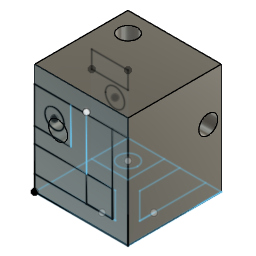
cornerpiece_test1 (Autodesk Fusion 360 design; units mm, degrees)
Autodesk Fusion 360 part; units mm, degrees
note: some values were not read from the file. Set by a fixed rule: which sketch regions a step uses.
sketch "Skizze1" plane through (0, 0, 0) normal (0, 0, 1) x (1, 0, 0)
  line L0 (4.1176, 5.2824) -> (204.1176, 5.2824)
  line L1 (204.1176, 5.2824) -> (204.1176, 205.2824)
  line L2 (204.1176, 205.2824) -> (4.1176, 205.2824)
  line L3 (4.1176, 205.2824) -> (4.1176, 5.2824)
  line L4 (204.1176, 48.8824) -> (207.3176, 48.8824)
  line L5 (207.3176, 48.8824) -> (207.3176, 13.2824)
  line L6 (207.3176, 13.2824) -> (204.1176, 13.2824)
  line L7 (204.1176, 13.2824) -> (204.1176, 48.8824)
  line L8 (196.1176, 13.2824) -> (207.1176, 13.2824)
  line L9 (207.1176, 13.2824) -> (207.1176, 2.2824)
  line L10 (207.1176, 2.2824) -> (196.1176, 2.2824)
  line L11 (196.1176, 2.2824) -> (196.1176, 13.2824)
  circle A0 centre (202.6176, 6.7824) radius 1
  line L12 (202.1176, 5.2824) -> (204.1176, 7.2824)
  dimension "top_w" = 200
  dimension "top_l" = 200
  dimension "d12" = 3.2
  dimension "d13" = 35.6
  dimension "d14" = 11
  dimension "d15" = 11
  dimension "d17" = 2
  dimension "d18" = 1.5
  dimension "d19" = 1.5
  dimension "d23" = 3
  dimension "d24" = 3
  dimension "d28" = 2
  dimension "d29" = 2
  constraint horizontal L0
  constraint vertical L1
  constraint horizontal L2
  constraint vertical L3
  constraint horizontal L4
  constraint vertical L5
  constraint horizontal L6
  constraint vertical L7
  constraint horizontal L8
  constraint vertical L9
  constraint horizontal L10
  constraint vertical L11
  constraint coincident L6.end L8
  constraint coincident L1 L6.end
  constraint coincident L0 L12.start
  constraint coincident L1 L12.end
  measures "top_w" distance of L0.start L0.end
  measures "top_l" distance of L0.start L2.end
  measures "d12" distance of L4.start L4.end
  measures "d13" distance of L4.start L6.end
  measures "d14" distance of L8.start L8.end
  measures "d15" distance of L8.start L10.end
  measures "d17" diameter of A0
  measures "d18" horizontal distance of L0.end A0.centre
  measures "d19" vertical distance of L0.end A0.centre
  measures "d23" horizontal distance of L0.end L9.end
  measures "d24" vertical distance of L0.end L9.end
  measures "d28" distance of L0.end L12.end
  measures "d29" distance of L0.end L12.start
sketch "Skizze2" plane through (0, 0, 0) normal (0, 0, 1) x (1, 0, 0)
  line L0 (17.1763, 11.0643) -> (17.1763, 0.2643)
  line L1 (6.3763, 0.2643) -> (6.3763, 11.0643)
  line L2 (6.3763, 11.0643) -> (17.1763, 11.0643)
  circle A0 centre (8.6763, 8.7643) radius 1.1
  line L3 (17.1763, 0.2643) -> (6.3763, 0.2643)
  line L4 (15.3763, 3.4319) -> (15.3763, 11.0643)
  line L5 (13.9155, 2.0643) -> (6.3763, 2.0643)
  line L6 (12.3763, 6.4319) -> (12.3763, 11.0643)
  line L7 (10.9155, 5.0643) -> (6.3763, 5.0643)
  line L8 (10.5763, 6.8643) -> (10.5763, 11.0643)
  line L9 (10.5763, 6.8643) -> (6.3763, 6.8643)
  line L10 (15.3763, 5.0643) -> (15.3763, 3.4319)
  line L11 (13.9155, 2.0643) -> (12.3763, 2.0643)
  line L12 (13.9155, 2.0643) -> (10.9155, 5.0643)
  line L13 (12.3763, 6.4319) -> (15.3763, 3.4319)
  dimension "d31" = 10.8
  dimension "d32" = 10.8
  dimension "d33" = 2.2
  dimension "sketch_screwhole_distx" = 8.5
  dimension "sketch_screwhole_disty" = 8.5
  dimension "d82" = 45
  dimension "d83" = 2
  dimension "d84" = 1.8
  dimension "d85" = 1.8
  dimension "d86" = 3
  dimension "d87" = 3
  constraint horizontal L2
  constraint vertical L0
  constraint horizontal L3
  constraint vertical L1
  constraint vertical L4
  constraint coincident L1 L5.end
  constraint perpendicular L1 L5
  constraint coincident L1 L7.end
  constraint perpendicular L1 L7
  constraint coincident L2 L8.end
  constraint coincident L1 L9.end
  constraint perpendicular L1 L9
  constraint coincident L2 L4.end
  constraint vertical L10
  constraint horizontal L11
  constraint parallel L12 L13
  constraint coincident L2 L6.end
  measures "d31" distance of L0.start L1.end
  measures "d32" distance of L1.end L1.start
  measures "d33" diameter of A0
  measures "sketch_screwhole_distx" horizontal distance of L0.end A0.centre
  measures "sketch_screwhole_disty" vertical distance of L0.end A0.centre
  measures "d82" angle of L7 L12
  measures "d83" distance of L12 L13
  measures "d84" distance of L3 L5.start
  measures "d85" distance of L0 L4.start
  measures "d86" distance of L5 L7
  measures "d87" distance of L4 L6
extrude "Extrusion1" add sketch "Skizze2" along normal blind 12.8 contours L0 L1 L2 L3 L4 L5 L6 L7 L8 L9 L10 L11 L12 L13 | L2 L4 L6 L10 L13 | L1 L5 L7 L11 L12 | L1 L2 L8 L9 | A0
extrude "Extrusion2" cut sketch "Skizze2" along normal blind 11 contours L2 L4 L6 L10 L13 | L1 L5 L7 L11 L12 | L1 L2 L8 L9
extrude "Extrusion3" cut sketch "Skizze2" along normal blind 12.8 contours A0
sketch "Skizze3" plane through (0, 0, 12.8) normal (0, 0, 1) x (-1, 0, 0)
  circle A0 centre (-8.6763, -8.7643) radius 1.1
  line L0 (-17.1763, -0.2643) -> (-17.1763, -11.0643)
  line L1 (-17.1763, -11.0643) -> (-6.3763, -11.0643)
  line L2 (-6.3763, -11.0643) -> (-6.3763, -0.2643)
  line L3 (-6.3763, -0.2643) -> (-17.1763, -0.2643)
sketch "Skizze4" plane through (0, 0.2643, 0) normal (0, -1, 0) x (1, 0, 0)
  line L0 (6.3763, 0) -> (17.1763, 0)
  line L1 (17.1763, 0) -> (17.1763, 12.8)
  line L2 (17.1763, 12.8) -> (6.3763, 12.8)
  line L3 (6.3763, 12.8) -> (6.3763, 0)
  line L4 (10.5763, 6.6) -> (10.5763, 10.8)
  line L5 (17.1763, 10.8) -> (17.1763, 0)
  line L6 (10.5763, 6.6) -> (6.3763, 6.6)
  line L7 (15.3763, 4.8) -> (15.3763, 1.8)
  circle A0 centre (8.6763, 8.5) radius 1.1
  line L8 (6.3763, 0) -> (6.3763, 10.8)
  line L9 (15.3763, 1.8) -> (6.3763, 1.8)
  line L10 (17.1763, 0) -> (6.3763, 0)
  line L11 (12.3763, 4.8) -> (15.3763, 4.8)
  line L12 (12.3763, 1.8) -> (12.3763, 4.8)
  line L13 (12.3763, 4.8) -> (12.3763, 11)
  line L14 (15.3763, 1.8) -> (15.3763, 10.8)
  line L15 (12.3763, 4.8) -> (6.3763, 4.8)
  line L16 (6.3763, 10.8) -> (17.1763, 10.8)
  line L17 (15.3763, 1.8) -> (12.3763, 1.8)
  dimension "d54" = 10.8
  dimension "d55" = 10.8
  dimension "d56" = 2.2
  dimension "d57" = 8.5
  dimension "d58" = 8.5
  dimension "d59" = 1.8
  dimension "d60" = 1.8
  dimension "d61" = 1.8
  dimension "d62" = 1.8
  dimension "d63" = 3
  dimension "d64" = 3
  constraint horizontal L16
  constraint vertical L5
  constraint horizontal L10
  constraint vertical L8
  constraint vertical L14
  constraint coincident L9.end L8
  constraint perpendicular L8 L9
  constraint coincident L15.end L8
  constraint perpendicular L8 L15
  constraint coincident L4.end L16
  constraint coincident L6.end L8
  constraint perpendicular L6 L8
  constraint coincident L14.end L16
  constraint horizontal L11
  constraint vertical L7
  constraint horizontal L17
  constraint vertical L12
  constraint coincident L0.start L3.end
  measures "d54" distance of L5.start L8.end
  measures "d55" distance of L0.start L8.end
  measures "d56" diameter of A0
  measures "d57" horizontal distance of A0.centre L0.end
  measures "d58" vertical distance of A0.centre L0.end
  measures "d59" vertical distance of L7.end L0.end
  measures "d60" horizontal distance of L7.end L0.end
  measures "d61" horizontal distance of L11.start L4.start
  measures "d62" vertical distance of L11.start L4.start
  measures "d63" vertical distance of L7.end L11.start
  measures "d64" horizontal distance of L7.end L11.start
sketch "Skizze5" plane through (0, 6.8643, 0) normal (0, 1, 0) x (-1, 0, 0)
  line L0 (-10.5763, 0) -> (-6.3763, 0)
  line L1 (-6.3763, 0) -> (-6.3763, 11)
  line L2 (-6.3763, 11) -> (-10.5763, 11)
  line L3 (-10.5763, 11) -> (-10.5763, 0)
  line L4 (-10.5763, 11) -> (-6.3763, 11)
  line L5 (-6.3763, 11) -> (-6.3763, 9)
  line L6 (-6.3763, 9) -> (-10.5763, 9)
  line L7 (-10.5763, 9) -> (-10.5763, 11)
  circle A0 centre (-9.0763, 7.5) radius 1.1
  dimension "front_topinset_height" = 2
  dimension "d70" = 2.2
  dimension "d71" = 1.5
  dimension "d72" = 1.5
  constraint horizontal L4
  constraint vertical L5
  constraint horizontal L6
  constraint vertical L7
  constraint coincident L1 L5.end
  constraint coincident L2.end L3.start
  measures "front_topinset_height" distance of L2.end L6.end
  measures "d70" diameter of A0
  measures "d71" horizontal distance of L6.end A0.centre
  measures "d72" vertical distance of L6.end A0.centre
extrude "Extrusion4" cut sketch "Skizze5" against normal blind 1.8 contours L1 L2 L3 L4 L5 L6 L7
sketch "Skizze6" plane through (10.5763, 0, 0) normal (-1, 0, 0) x (0, -1, 0)
  line L0 (-11.0643, 0) -> (-6.8643, 0)
  line L1 (-6.8643, 0) -> (-6.8643, 9)
  line L2 (-6.8643, 9) -> (-5.0643, 9)
  line L3 (-5.0643, 9) -> (-5.0643, 11)
  line L4 (-5.0643, 11) -> (-11.0643, 11)
  line L5 (-11.0643, 11) -> (-11.0643, 0)
  line L6 (-5.0643, 11) -> (-11.0643, 11)
  line L7 (-11.0643, 11) -> (-11.0643, 9)
  line L8 (-11.0643, 9) -> (-5.0643, 9)
  line L9 (-5.0643, 9) -> (-5.0643, 11)
  circle A0 centre (-9.5643, 7.5) radius 1.1
  dimension "d75" = 2.2
  dimension "d76" = 1.5
  dimension "d77" = 1.5
  constraint horizontal L6
  constraint vertical L7
  constraint horizontal L8
  constraint vertical L9
  constraint coincident L5 L7.end
  constraint coincident L3.end L4.start
  measures "d75" diameter of A0
  measures "d76" horizontal distance of L7.end A0.centre
  measures "d77" vertical distance of L7.end A0.centre
extrude "Extrusion6" cut sketch "Skizze5" against normal blind 7 contours A0
extrude "Extrusion7" cut sketch "Skizze6" against normal blind 7 contours A0
extrude "Extrusion8" cut sketch "Skizze6" against normal blind 1.8 contours L2 L3 L4 L5 L6 L7 L8 L9
sketch "Skizze7" plane through (0, 11.0643, 0) normal (0, 1, 0) x (-1, 0, 0)
  line L0 (-15.3763, 11) -> (-6.3763, 11)
  line L1 (-6.3763, 11) -> (-6.3763, 12.8)
  line L2 (-6.3763, 12.8) -> (-17.1763, 12.8)
  line L3 (-17.1763, 12.8) -> (-17.1763, 0)
  line L4 (-17.1763, 0) -> (-15.3763, 0)
  line L5 (-15.3763, 0) -> (-15.3763, 11)
  line L6 (-15.3763, 11) -> (-10.5, 11)
  line L7 (-10.5, 11) -> (-10.5, 9)
  line L8 (-10.5, 9) -> (-15.3763, 9)
  line L9 (-15.3763, 9) -> (-15.3763, 11)
  constraint horizontal L6
  constraint vertical L7
  constraint horizontal L8
  constraint vertical L9
  constraint coincident L0.start L5.end
extrude "Extrusion9" cut sketch "Skizze7" against normal blind 9 contours L0 L5 L6 L7 L8 L9
extrude "Extrusion5" [suppressed]
equation "inside_w = 200 mm"
equation "inside_h = 70 mm"
equation "inside_l = 200 mm"
equation "woodkerf = 0.2 mm"
equation "plastickerf = 0.2 mm"
equation "border_w = 5 mm"
equation "woodthickness = 3 mm"
equation "top_w = inside_w"
equation "top_l = inside_l"
equation "cornerjoint_w = 11 mm"
equation "screwhole_dist = screw_d * 0.75"
equation "d12 = woodkerf + woodthickness"
equation "d13 = ( top_l - ( 2 * cornerjoint_w ) ) / woodjointcount"
equation "d14 = cornerjoint_w"
equation "d15 = cornerjoint_w"
equation "screw_d = 2 mm"
equation "d17 = screw_d"
equation "d18 = screwhole_dist"
equation "d19 = screwhole_dist"
equation "cornerjoint_wall_thickness = 2 mm"
equation "d23 = woodthickness"
equation "d24 = woodthickness"
equation "woodjointcount = 5"
equation "bevel = 2 mm"
equation "d28 = bevel"
equation "d29 = bevel"
equation "feetheight = 10 mm"
equation "d31 = cornerjoint_w - plastickerf"
equation "d32 = cornerjoint_w - plastickerf"
equation "d33 = screw_d + plastickerf"
equation "sketch_screwhole_distx = ( 2 * cornerjoint_wall_thickness ) + woodthickness + screwhole_dist"
equation "sketch_screwhole_disty = ( 2 * cornerjoint_wall_thickness ) + woodthickness + screwhole_dist"
equation "base_corner_top = cornerjoint_w + cornerjoint_wall_thickness - plastickerf"
equation "neg_corner_top = cornerjoint_w"
equation "neg_screwhole_top = base_corner_top"
equation "d54 = cornerjoint_w - plastickerf"
equation "d55 = cornerjoint_w - plastickerf"
equation "d56 = screw_d + plastickerf"
equation "d57 = ( 2 * cornerjoint_wall_thickness ) + woodthickness + screwhole_dist"
equation "d58 = ( 2 * cornerjoint_wall_thickness ) + woodthickness + screwhole_dist"
equation "d59 = cornerjoint_wall_thickness - plastickerf"
equation "d60 = cornerjoint_wall_thickness - plastickerf"
equation "d61 = cornerjoint_wall_thickness - plastickerf"
equation "d62 = cornerjoint_wall_thickness - plastickerf"
equation "d63 = woodthickness"
equation "d64 = woodthickness"
equation "front_topinset_height = cornerjoint_wall_thickness"
equation "front_topinset_thickness = -( cornerjoint_wall_thickness - plastickerf )"
equation "d68 = -( cornerjoint_wall_thickness - plastickerf )"
equation "d70 = screw_d + plastickerf"
equation "d71 = screwhole_dist"
equation "d72 = screwhole_dist"
equation "neg_front_topinset_screwhole = -( ( 2 * cornerjoint_wall_thickness ) + woodthickness )"
equation "d75 = screw_d + plastickerf"
equation "d76 = screwhole_dist"
equation "d77 = screwhole_dist"
equation "d78 = -( ( 2 * cornerjoint_wall_thickness ) + woodthickness )"
equation "d80 = -( cornerjoint_wall_thickness - plastickerf )"
equation "d83 = cornerjoint_wall_thickness"
equation "d84 = cornerjoint_wall_thickness - plastickerf"
equation "d85 = cornerjoint_wall_thickness - plastickerf"
equation "d86 = woodthickness"
equation "d87 = woodthickness"
equation "neg_cornerinset = -( d32 - ( cornerjoint_wall_thickness - plastickerf ) )"
